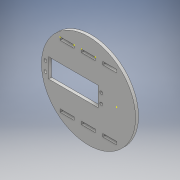
# Autodesk Inventor part: base2
Saved by Autodesk Inventor 2018 (Build 220112000, 112)
## iProperties
Created: 2020-03-10
Part Number: base2
Material: Genérico
Document SubType Name: Modeling
Designer: sala.ceri
Density: 1 g/cm^3
Appearance: Valor por defecto
Author: sala.ceri
Autodesk Inventor part; units mm, degrees
ref_plane "YZ Plane" through (0, 0, 0) normal (1, 0, 0) x (0, 1, 0)
ref_plane "XZ Plane" through (0, 0, 0) normal (0, 1, 0) x (-1, 0, 0)
ref_plane "XY Plane" through (0, 0, 0) normal (0, 0, 1) x (1, 0, 0)
sketch "Boceto1" plane through (0, 0, 0) normal (0, 1, 0) x (-1, 0, 0)
  circle A0 centre (28.5, 0) radius 1.5
  circle A1 centre (28.5, -8) radius 1.5
  circle A2 centre (28.5, 8) radius 1.5
  circle A3 centre (36.5, 0) radius 1.5
  circle A4 centre (20.5, 0) radius 1.5
  circle A5 centre (28.5, 0) radius 47.5
  line L0 (57, 33) -> (43, 33)
  line L1 (43, 33) -> (43, 30)
  line L2 (35.5, 30) -> (35.5, 33)
  line L3 (35.5, 33) -> (21.5, 33)
  line L4 (21.5, 33) -> (21.5, 30)
  line L5 (14, 30) -> (14, 33)
  line L6 (14, 33) -> (0, 33)
  line L7 (43, 30) -> (57, 30)
  line L8 (21.5, 30) -> (35.5, 30)
  line L9 (14, 30) -> (0, 30)
  line L10 (0, 30) -> (0, 33)
  line L11 (57, 33) -> (57, 30)
  line L12 (35.5, -30) -> (35.5, -33)
  line L13 (21.5, -30) -> (35.5, -30)
  line L14 (35.5, -33) -> (21.5, -33)
  line L15 (21.5, -33) -> (21.5, -30)
  line L16 (57, -33) -> (43, -33)
  line L17 (43, -33) -> (43, -30)
  line L18 (43, -30) -> (57, -30)
  line L19 (14, -30) -> (14, -33)
  line L20 (14, -30) -> (0, -30)
  line L21 (14, -33) -> (0, -33)
  line L22 (0, -30) -> (0, -33)
  line L23 (57, -33) -> (57, -30)
  constraints: 48 end point, 10 point on line, 6 centre point, 1 coincident, 1 vertical
extrude "Extrusión1" add sketch "Boceto1" along normal blind 3
sketch "Boceto2" plane through (-28.5, 0, 0) normal (0, -1, 0) x (1, 0, 0)
  circle A0 centre (0, 0) radius 3.5
  point P0 (28.5, 0)
  dimension "d23" = 7
  constraints: 1 centre point
  measures "d23" diameter of A0
extrude "Extrusión2" cut sketch "Boceto2" against normal blind 10
sketch "Boceto3" plane through (-28.5, 0, 0) normal (0, -1, 0) x (1, 0, 0)
  circle A0 centre (0, 0) radius 4.5
  point P0 (28.5, 0)
  dimension "d26" = 9
  constraints: 1 centre point
  measures "d26" diameter of A0
extrude "Extrusión3" cut sketch "Boceto3" against normal blind 10
sketch "Boceto4" plane through (-28.5, 0, 0) normal (0, -1, 0) x (1, 0, 0)
  line L0 (-40.25, 9.75) -> (9.75, 9.75)
  line L1 (9.75, 9.75) -> (9.75, -9.75)
  line L2 (9.75, -9.75) -> (-40.25, -9.75)
  line L3 (-40.25, -9.75) -> (-40.25, 9.75)
  circle A0 centre (-43.5, 4.875) radius 1.5
  circle A1 centre (-43.5, -4.875) radius 1.5
  circle A2 centre (13, 4.875) radius 1.5
  circle A3 centre (13, -4.875) radius 1.5
  point P0 (28.5, 0)
  point P1 (-28.5, 33)
  point P2 (28.5, 33)
  point P3 (28.5, 30)
  point P4 (-28.5, -33)
  point P5 (0, 0)
  dimension "d32" = 50
  constraints: 8 end point, 4 centre point, 2 perpendicular, 1 horizontal
  measures "d32" distance of L0.start L0.end
extrude "Extrusión4" cut sketch "Boceto4" against normal blind 3
sketch "Boceto5" plane through (-28.5, 0, 0) normal (0, -1, 0) x (1, 0, 0)
  point P0 (28.5, 0)
  point P1 (-14.5, 33)
  point P2 (-28.5, 33)
  point P3 (7, 33)
  point P4 (-7, 33)
